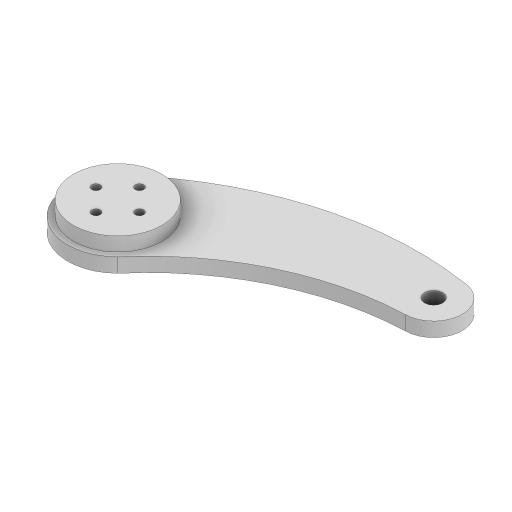
# Autodesk Inventor part: Link1V1R
Saved by Autodesk Inventor 2024.3 (Build 283343000, 343)
## iProperties
Created: 2025-10-01
Part Number: Link1V1R
Material: Generic
Document SubType Name: Modeling
Designer: danie
Density: 1 g/cm^3
Appearance: Default
Author: danie
Autodesk Inventor part; units mm, degrees
ref_plane "YZ Plane" through (0, 0, 0) normal (1, 0, 0) x (0, 1, 0)
ref_plane "XZ Plane" through (0, 0, 0) normal (0, 1, 0) x (-1, 0, 0)
ref_plane "XY Plane" through (0, 0, 0) normal (0, 0, 1) x (1, 0, 0)
sketch "Cara" plane through (0, 0, 0) normal (0, 0, 1) x (1, 0, 0)
  line L0 (-22.1935, -24.9393) -> (-15.1747, -17.9205)
  arc A0 (-12.474, -17.8034) -> (-15.1747, -17.9205) centre (-13.7605, -19.3347) ccw
  arc A1 (-12.474, -17.8034) -> (-6.107, -21.4794) centre (1.0981, -1.6477) ccw
  arc A2 (-4.8581, -23.8768) -> (-6.107, -21.4794) centre (-6.79, -23.3592) ccw
  line L1 (-4.8581, -23.8768) -> (-7.4272, -33.4646)
  arc A3 (-9.9928, -34.8439) -> (-7.4272, -33.4646) centre (-9.359, -32.947) ccw
  arc A4 (-22.1052, -27.8509) -> (-9.9928, -34.8439) centre (1.0981, -1.6477) ccw
  arc A5 (-22.1935, -24.9393) -> (-22.1052, -27.8509) centre (-20.7793, -26.3535) ccw
  line L2 (9.6235, -33.4646) -> (7.0544, -23.8768)
  arc A6 (8.3033, -21.4794) -> (7.0544, -23.8768) centre (8.9863, -23.3592) ccw
  arc A7 (8.3033, -21.4794) -> (14.6703, -17.8034) centre (1.0981, -1.6477) ccw
  arc A8 (17.371, -17.9205) -> (14.6703, -17.8034) centre (15.9568, -19.3347) ccw
  line L3 (17.371, -17.9205) -> (24.3898, -24.9393)
  arc A9 (24.3015, -27.8509) -> (24.3898, -24.9393) centre (22.9756, -26.3535) ccw
  arc A10 (12.1891, -34.8439) -> (24.3015, -27.8509) centre (1.0981, -1.6477) ccw
  arc A11 (9.6235, -33.4646) -> (12.1891, -34.8439) centre (11.5553, -32.947) ccw
  line L4 (32.9151, -10.173) -> (23.3272, -7.604)
  arc A12 (21.8755, -5.3237) -> (23.3272, -7.604) centre (23.8449, -5.6721) ccw
  arc A13 (21.8755, -5.3237) -> (21.8755, 2.0283) centre (1.0981, -1.6477) ccw
  arc A14 (23.3272, 4.3086) -> (21.8755, 2.0283) centre (23.8449, 2.3767) ccw
  line L5 (23.3272, 4.3086) -> (32.9151, 6.8776)
  arc A15 (35.3924, 5.3454) -> (32.9151, 6.8776) centre (33.4327, 4.9458) ccw
  arc A16 (35.3924, -8.6408) -> (35.3924, 5.3454) centre (1.0981, -1.6477) ccw
  arc A17 (32.9151, -10.173) -> (35.3924, -8.6408) centre (33.4327, -8.2412) ccw
  line L6 (24.3898, 21.6439) -> (17.371, 14.6251)
  arc A18 (14.6703, 14.508) -> (17.371, 14.6251) centre (15.9568, 16.0394) ccw
  arc A19 (14.6703, 14.508) -> (8.3033, 18.184) centre (1.0981, -1.6477) ccw
  arc A20 (7.0544, 20.5814) -> (8.3033, 18.184) centre (8.9863, 20.0638) ccw
  line L7 (7.0544, 20.5814) -> (9.6235, 30.1693)
  arc A21 (12.1891, 31.5486) -> (9.6235, 30.1693) centre (11.5553, 29.6516) ccw
  arc A22 (24.3015, 24.5555) -> (12.1891, 31.5486) centre (1.0981, -1.6477) ccw
  arc A23 (24.3898, 21.6439) -> (24.3015, 24.5555) centre (22.9756, 23.0582) ccw
  line L8 (-7.4272, 30.1693) -> (-4.8581, 20.5814)
  arc A24 (-6.107, 18.184) -> (-4.8581, 20.5814) centre (-6.79, 20.0638) ccw
  arc A25 (-6.107, 18.184) -> (-12.474, 14.508) centre (1.0981, -1.6477) ccw
  arc A26 (-15.1747, 14.6251) -> (-12.474, 14.508) centre (-13.7605, 16.0394) ccw
  line L9 (-15.1747, 14.6251) -> (-22.1935, 21.6439)
  arc A27 (-22.1052, 24.5555) -> (-22.1935, 21.6439) centre (-20.7793, 23.0582) ccw
  arc A28 (-9.9928, 31.5486) -> (-22.1052, 24.5555) centre (1.0981, -1.6477) ccw
  arc A29 (-7.4272, 30.1693) -> (-9.9928, 31.5486) centre (-9.359, 29.6516) ccw
  line L10 (-30.7188, 6.8776) -> (-21.131, 4.3086)
  arc A30 (-19.6792, 2.0283) -> (-21.131, 4.3086) centre (-21.6486, 2.3767) ccw
  arc A31 (-19.6792, 2.0283) -> (-19.6792, -5.3237) centre (1.0981, -1.6477) ccw
  arc A32 (-21.131, -7.604) -> (-19.6792, -5.3237) centre (-21.6486, -5.6721) ccw
  line L11 (-21.131, -7.604) -> (-30.7188, -10.173)
  arc A33 (-33.1961, -8.6408) -> (-30.7188, -10.173) centre (-31.2365, -8.2412) ccw
  arc A34 (-33.1961, 5.3454) -> (-33.1961, -8.6408) centre (1.0981, -1.6477) ccw
  arc A35 (-30.7188, 6.8776) -> (-33.1961, 5.3454) centre (-31.2365, 4.9458) ccw
  circle A36 centre (-37.4568, -19.3542) radius 1.5875
  circle A37 centre (39.653, 16.0588) radius 1.5875
  circle A38 centre (-16.6083, 36.9072) radius 1.5875
  circle A39 centre (18.8046, -40.2026) radius 1.5875
  circle A40 centre (1.0981, -1.6477) radius 15.5
  arc A41 (13.186, 39.6183) -> (16.9444, 39.4394) centre (15.4349, 47.2957) ccw
  arc A42 (13.186, 39.6183) -> (-10.9897, 39.6183) centre (1.0981, -1.6477) ccw
  arc A43 (-15.0916, 39.5133) -> (-10.9897, 39.6183) centre (-13.2386, 47.2957) ccw
  arc A44 (-15.0916, 39.5133) -> (-19.5734, 37.455) centre (-16.0181, 35.6221) ccw
  arc A45 (-22.3261, 34.412) -> (-19.5734, 37.455) centre (-26.6841, 41.1208) ccw
  arc A46 (-22.3261, 34.412) -> (-34.8255, 21.9848) centre (1.0981, -1.6477) ccw
  arc A47 (-37.5746, 19.4158) -> (-34.8255, 21.9848) centre (-41.5089, 26.3816) ccw
  arc A48 (-39.989, 14.1986) -> (-37.5746, 19.4158) centre (-37.4054, 16.1703) ccw
  arc A49 (-40.1679, 10.4402) -> (-39.989, 14.1986) centre (-47.8453, 12.6891) ccw
  arc A50 (-40.1679, 10.4402) -> (-40.2027, -13.6161) centre (1.0981, -1.6477) ccw
  arc A51 (-40.1338, -17.8165) -> (-40.2027, -13.6161) centre (-47.8865, -15.8428) ccw
  arc A52 (-40.1338, -17.8165) -> (-38.0349, -22.3868) centre (-36.2575, -18.8034) ccw
  arc A53 (-34.8937, -25.1762) -> (-38.0349, -22.3868) centre (-41.5898, -29.5536) ccw
  arc A54 (-34.8937, -25.1762) -> (-22.5344, -37.5713) centre (1.0981, -1.6477) ccw
  arc A55 (-19.9654, -40.3204) -> (-22.5344, -37.5713) centre (-26.9311, -44.2547) ccw
  arc A56 (-14.7481, -42.7348) -> (-19.9654, -40.3204) centre (-16.7198, -40.1512) ccw
  arc A57 (-10.9897, -42.9137) -> (-14.7481, -42.7348) centre (-13.2386, -50.5911) ccw
  arc A58 (-10.9897, -42.9137) -> (13.0666, -42.9485) centre (1.0981, -1.6477) ccw
  arc A59 (17.2235, -42.8687) -> (13.0666, -42.9485) centre (15.2932, -50.6324) ccw
  arc A60 (17.2235, -42.8687) -> (21.7574, -40.7935) centre (18.1887, -38.9869) ccw
  arc A61 (24.5347, -37.6994) -> (21.7574, -40.7935) centre (28.895, -44.4067) ccw
  arc A62 (24.5347, -37.6994) -> (37.0217, -25.2802) centre (1.0981, -1.6477) ccw
  arc A63 (39.7709, -22.7112) -> (37.0217, -25.2802) centre (43.7052, -29.6769) ccw
  arc A64 (42.1093, -17.3982) -> (39.7709, -22.7112) centre (39.6017, -19.4656) ccw
  arc A65 (42.3332, -13.8408) -> (42.1093, -17.3982) centre (50.0048, -16.1093) ccw
  arc A66 (42.3332, -13.8408) -> (42.3989, 10.3207) centre (1.0981, -1.6477) ccw
  arc A67 (42.3301, 14.5211) -> (42.3989, 10.3207) centre (50.0828, 12.5474) ccw
  arc A68 (42.3301, 14.5211) -> (40.2312, 19.0914) centre (38.4538, 15.508) ccw
  arc A69 (37.09, 21.8808) -> (40.2312, 19.0914) centre (43.7861, 26.2582) ccw
  arc A70 (37.09, 21.8808) -> (24.7307, 34.2759) centre (1.0981, -1.6477) ccw
  arc A71 (22.1617, 37.0251) -> (24.7307, 34.2759) centre (29.1274, 40.9594) ccw
  arc A72 (16.9444, 39.4394) -> (22.1617, 37.0251) centre (18.9161, 36.8558) ccw
  arc A73 (-38.8583, 20.9988) -> (-42.0265, 14.1525) centre (-36.2077, 15.616) ccw
  spline S0 degree 3 poles (-40.2504, 14.5992) (-40.3671, 14.8104) (-40.4601, 15.0344) (-40.6458, 15.6766) (-40.6826, 16.1053) (-40.5958, 16.8869) (-40.4968, 17.2357) (-40.1864, 17.8912) (-39.9757, 18.1925) (-39.4148, 18.7612) (-39.0515, 19.0059) (-38.4565, 19.2528) (-38.255, 19.3143) (-38.0493, 19.3558) knots 0 0 0 0 0.118944 0.118944 0.328096 0.328096 0.504735 0.504735 0.683825 0.683825 0.89662 0.89662 1 1 1 1
  line L12 (-38.8583, 20.9988) -> (-38.0493, 19.3558)
  arc A74 (-38.8583, 20.9988) -> (-42.0265, 14.1525) centre (-36.2077, 15.616) ccw
  line L13 (-40.2504, 14.5992) -> (-42.0265, 14.1525)
  line L14 (-38.5582, 21.1573) -> (-37.5746, 19.4158)
  arc A75 (-37.5746, 19.4158) -> (-34.8255, 21.9848) centre (-41.5089, 26.3816) ccw
  line L15 (-36.4963, 23.084) -> (-34.8255, 21.9848)
  arc A76 (-38.5582, 21.1573) -> (-36.4963, 23.084) centre (-41.5089, 26.3816) ccw
  spline S1 degree 3 poles (-38.0493, 19.3558) (-37.9271, 19.3805) (-37.8093, 19.397) (-37.6564, 19.4108) (-37.6155, 19.4137) (-37.5746, 19.4158) knots 0 0 0 0 0.731153 0.731153 1 1 1 1
  line L16 (-38.5582, 21.1573) -> (-37.5746, 19.4158)
  arc A77 (-38.8583, 20.9988) -> (-38.5582, 21.1573) centre (-41.5089, 26.3816) ccw
  line L17 (-38.8583, 20.9988) -> (-38.0493, 19.3558)
  spline S2 degree 3 poles (-39.989, 14.1986) (-40.081, 14.3191) (-40.1695, 14.4526) (-40.2504, 14.5992) knots 0 0 0 0 1 1 1 1
  line L18 (-40.2504, 14.5992) -> (-42.0265, 14.1525)
  arc A78 (-41.953, 13.8212) -> (-42.0265, 14.1525) centre (-47.8453, 12.6891) ccw
  line L19 (-39.989, 14.1986) -> (-41.953, 13.8212)
  line L20 (-39.989, 14.1986) -> (-41.953, 13.8212)
  arc A79 (-42.0872, 11.0024) -> (-41.953, 13.8212) centre (-47.8453, 12.6891) ccw
  line L21 (-42.0872, 11.0024) -> (-40.1679, 10.4402)
  arc A80 (-40.1679, 10.4402) -> (-39.989, 14.1986) centre (-47.8453, 12.6891) ccw
  arc A81 (-42.0872, 11.0024) -> (-42.1236, -14.1728) centre (1.0981, -1.6477) ccw
  line L22 (-36.4963, 23.084) -> (-34.8255, 21.9848)
  arc A82 (-22.3261, 34.412) -> (-34.8255, 21.9848) centre (1.0981, -1.6477) ccw
  line L23 (-23.4156, 36.0892) -> (-22.3261, 34.412)
  arc A83 (-23.4156, 36.0892) -> (-36.4963, 23.084) centre (1.0981, -1.6477) ccw
  line L24 (-23.4156, 36.0892) -> (-22.3261, 34.412)
  arc A84 (-22.3261, 34.412) -> (-19.5734, 37.455) centre (-26.6841, 41.1208) ccw
  line L25 (-21.3511, 38.3714) -> (-19.5734, 37.455)
  arc A85 (-23.4156, 36.0892) -> (-21.3511, 38.3714) centre (-26.6841, 41.1208) ccw
  line L26 (-21.3511, 38.3714) -> (-19.5734, 37.455)
  arc A86 (-15.0916, 39.5133) -> (-19.5734, 37.455) centre (-16.0181, 35.6221) ccw
  line L27 (-14.6284, 41.4589) -> (-15.0916, 39.5133)
  arc A87 (-14.6284, 41.4589) -> (-21.3511, 38.3714) centre (-16.0181, 35.6221) ccw
  line L28 (-14.6284, 41.4589) -> (-15.0916, 39.5133)
  arc A88 (-15.0916, 39.5133) -> (-10.9897, 39.6183) centre (-13.2386, 47.2957) ccw
  line L29 (-11.5519, 41.5377) -> (-10.9897, 39.6183)
  arc A89 (-14.6284, 41.4589) -> (-11.5519, 41.5377) centre (-13.2386, 47.2957) ccw
  line L30 (-11.5519, 41.5377) -> (-10.9897, 39.6183)
  arc A90 (13.186, 39.6183) -> (-10.9897, 39.6183) centre (1.0981, -1.6477) ccw
  line L31 (13.7482, 41.5377) -> (13.186, 39.6183)
  arc A91 (13.7482, 41.5377) -> (-11.5519, 41.5377) centre (1.0981, -1.6477) ccw
  line L32 (16.9444, 39.4394) -> (16.567, 41.4035)
  arc A92 (13.7482, 41.5377) -> (16.567, 41.4035) centre (15.4349, 47.2957) ccw
  line L33 (13.7482, 41.5377) -> (13.186, 39.6183)
  arc A93 (13.186, 39.6183) -> (16.9444, 39.4394) centre (15.4349, 47.2957) ccw
  spline S3 degree 3 poles (16.9444, 39.4394) (17.0649, 39.5314) (17.1985, 39.6199) (17.3451, 39.7009) knots 0 0 0 0 1 1 1 1
  line L34 (17.3451, 39.7009) -> (16.8984, 41.4769)
  arc A94 (16.567, 41.4035) -> (16.8984, 41.4769) centre (15.4349, 47.2957) ccw
  line L35 (16.9444, 39.4394) -> (16.567, 41.4035)
  spline S4 degree 3 poles (17.3451, 39.7009) (17.5563, 39.8175) (17.7803, 39.9105) (18.4224, 40.0962) (18.8512, 40.133) (19.6327, 40.0462) (19.9815, 39.9473) (20.6371, 39.6368) (20.9383, 39.4261) (21.507, 38.8652) (21.7517, 38.502) (21.9986, 37.907) (22.0601, 37.7054) (22.1017, 37.4997) knots 0 0 0 0 0.118944 0.118944 0.328096 0.328096 0.504735 0.504735 0.683825 0.683825 0.89662 0.89662 1 1 1 1
  line L36 (23.7446, 38.3088) -> (22.1017, 37.4997)
  arc A95 (23.7446, 38.3088) -> (16.8984, 41.4769) centre (18.3618, 35.6581) ccw
  line L37 (17.3451, 39.7009) -> (16.8984, 41.4769)
  line L38 (37.09, 21.8808) -> (38.764, 22.9751)
  arc A96 (38.764, 22.9751) -> (25.8298, 35.9468) centre (1.0981, -1.6477) ccw
  line L39 (25.8298, 35.9468) -> (24.7307, 34.2759)
  arc A97 (37.09, 21.8808) -> (24.7307, 34.2759) centre (1.0981, -1.6477) ccw
  line L40 (23.9031, 38.0086) -> (22.1617, 37.0251)
  arc A98 (22.1617, 37.0251) -> (24.7307, 34.2759) centre (29.1274, 40.9594) ccw
  line L41 (25.8298, 35.9468) -> (24.7307, 34.2759)
  arc A99 (23.9031, 38.0086) -> (25.8298, 35.9468) centre (29.1274, 40.9594) ccw
  spline S5 degree 3 poles (22.1017, 37.4997) (22.1264, 37.3775) (22.1428, 37.2598) (22.1566, 37.1069) (22.1595, 37.0659) (22.1617, 37.0251) knots 0 0 0 0 0.731153 0.731153 1 1 1 1
  line L42 (23.9031, 38.0086) -> (22.1617, 37.0251)
  arc A100 (23.7446, 38.3088) -> (23.9031, 38.0086) centre (29.1274, 40.9594) ccw
  line L43 (23.7446, 38.3088) -> (22.1017, 37.4997)
  line L44 (37.09, 21.8808) -> (38.764, 22.9751)
  arc A101 (37.09, 21.8808) -> (40.2312, 19.0914) centre (43.7861, 26.2582) ccw
  line L45 (41.1199, 20.8831) -> (40.2312, 19.0914)
  arc A102 (38.764, 22.9751) -> (41.1199, 20.8831) centre (43.7861, 26.2582) ccw
  line L46 (41.1199, 20.8831) -> (40.2312, 19.0914)
  arc A103 (42.3301, 14.5211) -> (40.2312, 19.0914) centre (38.4538, 15.508) ccw
  line L47 (44.2683, 14.0277) -> (42.3301, 14.5211)
  arc A104 (44.2683, 14.0277) -> (41.1199, 20.8831) centre (38.4538, 15.508) ccw
  line L48 (44.2683, 14.0277) -> (42.3301, 14.5211)
  arc A105 (42.3301, 14.5211) -> (42.3989, 10.3207) centre (50.0828, 12.5474) ccw
  line L49 (44.3199, 10.8774) -> (42.3989, 10.3207)
  arc A106 (44.2683, 14.0277) -> (44.3199, 10.8774) centre (50.0828, 12.5474) ccw
  line L50 (44.3199, 10.8774) -> (42.3989, 10.3207)
  arc A107 (42.3332, -13.8408) -> (42.3989, 10.3207) centre (1.0981, -1.6477) ccw
  line L51 (44.2511, -14.4079) -> (42.3332, -13.8408)
  arc A108 (44.2511, -14.4079) -> (44.3199, 10.8774) centre (1.0981, -1.6477) ccw
  spline S6 degree 3 poles (42.4708, -17.939) (42.66, -18.2947) (42.7816, -18.6826) (42.8764, -19.4825) (42.8492, -19.8873) (42.6667, -20.5952) (42.5369, -20.899) (42.1389, -21.5409) (41.845, -21.8556) (41.1886, -22.3275) (40.8415, -22.494) (40.3834, -22.6216) (40.2925, -22.6427) (40.2009, -22.6599) knots 0 0 0 0 0.198107 0.198107 0.395669 0.395669 0.556952 0.556952 0.766408 0.766408 0.954091 0.954091 1 1 1 1
  line L52 (41.0245, -24.3091) -> (40.2009, -22.6599)
  arc A109 (41.0245, -24.3091) -> (44.1743, -17.5253) centre (38.3438, -18.9413) ccw
  line L53 (42.4708, -17.939) -> (44.1743, -17.5253)
  line L54 (42.1093, -17.3982) -> (44.0832, -17.076)
  arc A110 (44.2511, -14.4079) -> (44.0832, -17.076) centre (50.0048, -16.1093) ccw
  line L55 (44.2511, -14.4079) -> (42.3332, -13.8408)
  arc A111 (42.3332, -13.8408) -> (42.1093, -17.3982) centre (50.0048, -16.1093) ccw
  spline S7 degree 3 poles (42.1093, -17.3982) (42.1251, -17.4173) (42.1406, -17.4367) (42.2692, -17.6002) (42.376, -17.7609) (42.4708, -17.939) knots 0 0 0 0 0.119683 0.119683 1 1 1 1
  line L56 (42.4708, -17.939) -> (44.1743, -17.5253)
  arc A112 (44.0832, -17.076) -> (44.1743, -17.5253) centre (50.0048, -16.1093) ccw
  line L57 (42.1093, -17.3982) -> (44.0832, -17.076)
  spline S8 degree 3 poles (40.2009, -22.6599) (40.0946, -22.6799) (39.9919, -22.6936) (39.8527, -22.7062) (39.8117, -22.7091) (39.7709, -22.7112) knots 0 0 0 0 0.704713 0.704713 1 1 1 1
  line L58 (40.7545, -24.4527) -> (39.7709, -22.7112)
  arc A113 (41.0245, -24.3091) -> (40.7545, -24.4527) centre (43.7052, -29.6769) ccw
  line L59 (41.0245, -24.3091) -> (40.2009, -22.6599)
  line L60 (40.7545, -24.4527) -> (39.7709, -22.7112)
  arc A114 (39.7709, -22.7112) -> (37.0217, -25.2802) centre (43.7052, -29.6769) ccw
  line L61 (38.6926, -26.3794) -> (37.0217, -25.2802)
  arc A115 (40.7545, -24.4527) -> (38.6926, -26.3794) centre (43.7052, -29.6769) ccw
  line L62 (38.6926, -26.3794) -> (37.0217, -25.2802)
  arc A116 (24.5347, -37.6994) -> (37.0217, -25.2802) centre (1.0981, -1.6477) ccw
  line L63 (25.6248, -39.3763) -> (24.5347, -37.6994)
  arc A117 (25.6248, -39.3763) -> (38.6926, -26.3794) centre (1.0981, -1.6477) ccw
  line L64 (25.6248, -39.3763) -> (24.5347, -37.6994)
  arc A118 (24.5347, -37.6994) -> (21.7574, -40.7935) centre (28.895, -44.4067) ccw
  line L65 (23.5418, -41.6968) -> (21.7574, -40.7935)
  arc A119 (25.6248, -39.3763) -> (23.5418, -41.6968) centre (28.895, -44.4067) ccw
  line L66 (23.5418, -41.6968) -> (21.7574, -40.7935)
  arc A120 (17.2235, -42.8687) -> (21.7574, -40.7935) centre (18.1887, -38.9869) ccw
  line L67 (16.7409, -44.8096) -> (17.2235, -42.8687)
  arc A121 (16.7409, -44.8096) -> (23.5418, -41.6968) centre (18.1887, -38.9869) ccw
  line L68 (16.7409, -44.8096) -> (17.2235, -42.8687)
  arc A122 (17.2235, -42.8687) -> (13.0666, -42.9485) centre (15.2932, -50.6324) ccw
  line L69 (13.6232, -44.8695) -> (13.0666, -42.9485)
  arc A123 (16.7409, -44.8096) -> (13.6232, -44.8695) centre (15.2932, -50.6324) ccw
  arc A124 (-10.9897, -42.9137) -> (13.0666, -42.9485) centre (1.0981, -1.6477) ccw
  line L70 (13.6232, -44.8695) -> (13.0666, -42.9485)
  arc A125 (-10.9897, -42.9137) -> (13.0666, -42.9485) centre (1.0981, -1.6477) ccw
  line L71 (-11.5519, -44.8331) -> (-10.9897, -42.9137)
  arc A126 (-11.5519, -44.8331) -> (13.6232, -44.8695) centre (1.0981, -1.6477) ccw
  line L72 (-14.7481, -42.7348) -> (-14.3707, -44.6989)
  arc A127 (-11.5519, -44.8331) -> (-14.3707, -44.6989) centre (-13.2386, -50.5911) ccw
  line L73 (-11.5519, -44.8331) -> (-10.9897, -42.9137)
  arc A128 (-10.9897, -42.9137) -> (-14.7481, -42.7348) centre (-13.2386, -50.5911) ccw
  spline S9 degree 3 poles (-15.1488, -42.9963) (-15.36, -43.1129) (-15.584, -43.2059) (-16.2261, -43.3916) (-16.6549, -43.4284) (-17.4365, -43.3416) (-17.7852, -43.2427) (-18.4408, -42.9322) (-18.742, -42.7215) (-19.3107, -42.1606) (-19.5554, -41.7973) (-19.8023, -41.2024) (-19.8638, -41.0008) (-19.9054, -40.7951) knots 0 0 0 0 0.118944 0.118944 0.328096 0.328096 0.504735 0.504735 0.683825 0.683825 0.89662 0.89662 1 1 1 1
  line L74 (-21.5483, -41.6041) -> (-19.9054, -40.7951)
  arc A129 (-21.5483, -41.6041) -> (-14.7021, -44.7723) centre (-16.1656, -38.9535) ccw
  line L75 (-15.1488, -42.9963) -> (-14.7021, -44.7723)
  spline S10 degree 3 poles (-14.7481, -42.7348) (-14.8686, -42.8268) (-15.0022, -42.9153) (-15.1488, -42.9963) knots 0 0 0 0 1 1 1 1
  line L76 (-15.1488, -42.9963) -> (-14.7021, -44.7723)
  arc A130 (-14.3707, -44.6989) -> (-14.7021, -44.7723) centre (-13.2386, -50.5911) ccw
  line L77 (-14.7481, -42.7348) -> (-14.3707, -44.6989)
  spline S11 degree 3 poles (-19.9054, -40.7951) (-19.9301, -40.6729) (-19.9466, -40.5552) (-19.9604, -40.4023) (-19.9633, -40.3613) (-19.9654, -40.3204) knots 0 0 0 0 0.731153 0.731153 1 1 1 1
  line L78 (-21.7068, -41.304) -> (-19.9654, -40.3204)
  arc A131 (-21.5483, -41.6041) -> (-21.7068, -41.304) centre (-26.9311, -44.2547) ccw
  line L79 (-21.5483, -41.6041) -> (-19.9054, -40.7951)
  circle A132 centre (-16.7198, -40.1512) radius 3.25
  circle A133 centre (-16.7198, -40.1512) radius 1.5875
  circle A134 centre (39.6017, -19.4656) radius 3.25
  circle A135 centre (39.6017, -19.4656) radius 1.5875
  circle A136 centre (18.9161, 36.8558) radius 3.25
  circle A137 centre (18.9161, 36.8558) radius 1.5875
  circle A138 centre (-37.4054, 16.1703) radius 3.25
  circle A139 centre (-37.4054, 16.1703) radius 1.5875
  line L80 (-42.072, -17.3231) -> (-40.1338, -17.8165)
  arc A140 (-40.1338, -17.8165) -> (-40.2027, -13.6161) centre (-47.8865, -15.8428) ccw
  line L81 (-42.1236, -14.1728) -> (-40.2027, -13.6161)
  arc A141 (-42.072, -17.3231) -> (-42.1236, -14.1728) centre (-47.8865, -15.8428) ccw
  line L82 (-38.9237, -24.1785) -> (-38.0349, -22.3868)
  arc A142 (-40.1338, -17.8165) -> (-38.0349, -22.3868) centre (-36.2575, -18.8034) ccw
  line L83 (-42.072, -17.3231) -> (-40.1338, -17.8165)
  arc A143 (-42.072, -17.3231) -> (-38.9237, -24.1785) centre (-36.2575, -18.8034) ccw
  line L84 (-36.5677, -26.2705) -> (-34.8937, -25.1762)
  arc A144 (-34.8937, -25.1762) -> (-38.0349, -22.3868) centre (-41.5898, -29.5536) ccw
  line L85 (-38.9237, -24.1785) -> (-38.0349, -22.3868)
  arc A145 (-36.5677, -26.2705) -> (-38.9237, -24.1785) centre (-41.5898, -29.5536) ccw
  line L86 (-23.6336, -39.2421) -> (-22.5344, -37.5713)
  arc A146 (-34.8937, -25.1762) -> (-22.5344, -37.5713) centre (1.0981, -1.6477) ccw
  line L87 (-36.5677, -26.2705) -> (-34.8937, -25.1762)
  arc A147 (-36.5677, -26.2705) -> (-23.6336, -39.2421) centre (1.0981, -1.6477) ccw
  line L88 (-21.7068, -41.304) -> (-19.9654, -40.3204)
  arc A148 (-19.9654, -40.3204) -> (-22.5344, -37.5713) centre (-26.9311, -44.2547) ccw
  line L89 (-23.6336, -39.2421) -> (-22.5344, -37.5713)
  arc A149 (-21.7068, -41.304) -> (-23.6336, -39.2421) centre (-26.9311, -44.2547) ccw
  point P0 (1.3022, -1.7009)
  dimension "d1" = 30
  dimension "d2" = 40
  dimension "d3" = 70
  dimension "d4" = 90
  dimension "d5" = 65
  dimension "d6" = 95
  dimension "d7" = 100
  dimension "d8" = 72
  dimension "d9" = 17
  dimension "d10" = 110
  dimension "d11" = 4
sketch "Sketch1" plane through (0, 0, 0) normal (0, 1, 0) x (-1, 0, 0)
  line L0 (124.1031, 264.7872) -> (124.1031, -182.5054) construction
  line L1 (124.1031, -182.5054) -> (-344.0995, -182.5054) construction
  line L2 (-344.0995, -182.5054) -> (-344.0995, 264.7872) construction
  line L3 (-344.0995, 264.7872) -> (124.1031, 264.7872) construction
  circle A0 centre (0, 0) radius 50
  circle A1 centre (0, 0) radius 17.5
  line L4 (0, 0) -> (-80, -30.4436)
  line L5 (0, 0) -> (0, -17.5)
  line L6 (0, 0) -> (-17.5, 0)
  circle A2 centre (-80, -30.4436) radius 10
  line L7 (0, 0) -> (12.3744, -12.3744)
  line L8 (-80, -30.4436) -> (-80, -40.4436)
  line L9 (-80, -30.4436) -> (-72.9289, -37.5146)
  arc A3 (-80, -40.4436) -> (12.3744, -12.3744) centre (-63.3574, 70.821) ccw
  line L10 (-80, -30.4436) -> (-80, -20.4436)
  line L11 (0, 0) -> (-12.3744, 12.3744)
  arc A4 (-80, -20.4436) -> (-12.3744, 12.3744) centre (-83.4964, 72.8458) ccw
  circle A5 centre (0, 0) radius 7.6
  circle A6 centre (7.6, 0) radius 1.5
  circle A7 centre (0, 7.6) radius 1.5
  circle A8 centre (-7.6, 0) radius 1.5
  circle A9 centre (0, -7.6) radius 1.5
  circle A10 centre (-80, -30.4436) radius 1.5
  dimension "d68" = 15.2
  dimension "d44" = 100
  dimension "d55" = 35
  dimension "d56" = 80
  dimension "d65" = 20
  dimension "d66" = 45
  dimension "d67" = 45
  dimension "d69" = 3
  dimension "d72" = 360
  dimension "d80" = 3
  constraints: 16 end point, 11 point on circle, 10 centre point, 4 coincident, 3 vertical, 1 horizontal, 1 horizontal alignment, 1 point on line, 13 other
  measures "d44" diameter of A0
  measures "d55" diameter of A1
  measures "d56" horizontal distance of L4.end A0.centre
  measures "d65" diameter of A2
  measures "d66" angle of L5 L7
  measures "d67" angle of L8 L9
  measures "d69" diameter of A6
  measures "d80" diameter of A10
extrude "Extrusion1" add sketch "Sketch1" along normal blind 5 contours A4 A1 L4 A0 | A0 L4 A2 A4 | A3 A2 L4 A0 | A0 L4 A1 A3 | L10 A10 L8 A2 | A2 L4 A10 L10 | A4 L11 A5 A8 L6 A1 | L8 A10 L9 A2 | A1 L5 A9 A5 L7 A3 | L4 A5 A9 L5 A1 | A1 L6 A8 A5 L4 | A2 L9 A10 L4 | A10 L4 L10 | L10 L8 A10 | A1 L7 A5 A6 A7 L11 | L8 L9 A10 | A5 A8 L6 L4 | L4 L5 A9 A5 | A10 L9 L4 | A5 A7 A6 L7 L11 | L11 L6 A8 A5 | A5 A9 L5 L7
sketch "Sketch2" plane through (0, 0, 0) normal (0, -1, 0) x (1, 0, 0)
  circle A0 centre (0, 0) radius 15.5
  circle A1 centre (-7.6, 0) radius 1.5 projected
  circle A2 centre (0, -7.6) radius 1.5 projected
  circle A3 centre (7.6, 0) radius 1.5 projected
  circle A4 centre (0, 7.6) radius 1.5 projected
  dimension "d77" = 31
  constraints: 1 centre point, 1 coincident
  measures "d77" diameter of A0
extrude "Extrusion2" add sketch "Sketch2" against normal blind 9.9
hole "Hole1" at (80, 0, -30.4436) direction (0, 1, 0) diameter 6.35 end through all
body "Solid1"
